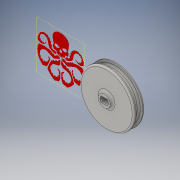
# Autodesk Inventor part: Wheel
Saved by Autodesk Inventor 2016 (Build 200138000, 138)
## iProperties
Created: 2017-09-08
Part Number: Wheel
Material: Generic
Document SubType Name: Modeling
Designer: student
Density: 1 g/cm^3
Appearance: Default
Author: student
Autodesk Inventor part; units mm, degrees
ref_plane "YZ Plane" through (0, 0, 0) normal (1, 0, 0) x (0, 1, 0)
ref_plane "XZ Plane" through (0, 0, 0) normal (0, 1, 0) x (-1, 0, 0)
ref_plane "XY Plane" through (0, 0, 0) normal (0, 0, 1) x (1, 0, 0)
sketch "Sketch8" plane through (0, 0, 0) normal (0, 0, 1) x (1, 0, 0)
  circle A0 centre (0, 0) radius 4.953
  dimension "d46" = 9.906
  constraints: 1 centre point, 1 coincident
  measures "d46" diameter of A0
extrude "Extrusion5" add sketch "Sketch8" along normal blind 2.032
sketch "Sketch9" plane through (0, 0, 0) normal (0, 0, -1) x (-1, 0, 0)
  circle A0 centre (0, 0) radius 22.479
  dimension "d49" = 44.958
  constraints: 1 centre point, 1 coincident
  measures "d49" diameter of A0
extrude "Extrusion6" add sketch "Sketch9" along normal blind 2.032
sketch "Sketch10" plane through (0, 0, -2.032) normal (0, 0, -1) x (-1, 0, 0)
  circle A0 centre (0, 0) radius 19.2405
  dimension "d52" = 38.481
  constraints: 1 centre point, 1 coincident
  measures "d52" diameter of A0
extrude "Extrusion7" add sketch "Sketch10" along normal blind 5.3086
sketch "Sketch11" plane through (0, 0, -7.3406) normal (0, 0, -1) x (-1, 0, 0)
  circle A0 centre (0, 0) radius 22.479
  dimension "d55" = 44.958
  constraints: 1 centre point, 1 coincident
  measures "d55" diameter of A0
extrude "Extrusion8" add sketch "Sketch11" along normal blind 2.032
fillet "Fillet1" radius 1.27 2 edges at (19.2405, 0, -2.032) (19.2405, 0, -7.3406)
sketch "Sketch12" plane through (0, 0, 2.032) normal (0, 0, 1) x (1, 0, 0)
  line L0 (2.5424, 2.413) -> (-2.5424, 2.413)
  line L1 (-2.5424, -2.413) -> (2.5424, -2.413)
  arc A0 (2.5424, -2.413) -> (2.5424, 2.413) centre (0, 0) ccw
  arc A1 (-2.5424, 2.413) -> (-2.5424, -2.413) centre (0, 0) ccw
  constraints: 4 end point, 4 point on circle, 2 centre point, 1 coincident, 1 horizontal, 1 parallel
fillet "Fillet2" radius 2.032 1 edges at (-4.953, 0, 0)
extrude "Extrusion9" cut sketch "Sketch12" against normal blind 5.4864
fillet "Fillet3" radius 1.27 2 edges at (22.479, 0, 0) (22.479, 0, -9.3726)
sketch "Sketch13" plane through (0, 0, -9.3726) normal (0, 0, -1) x (-1, 0, 0)
  line L0 (27.3817, 21.0767) -> (67.4327, 21.0767) construction
  line L1 (67.4327, 21.0767) -> (67.4327, -18.9549) construction
  line L2 (67.4327, -18.9549) -> (27.3817, -18.9549) construction
  line L3 (27.3817, -18.9549) -> (27.3817, 21.0767) construction
  point P0 (0, 0)
  constraints: 2 other
sketch "Sketch14" plane through (0, 0, -9.3726) normal (0, 0, -1) x (-1, 0, 0)
  arc A0 (-4.5923, 12.1139) -> (-4.8812, 11.9177) centre (-4.2357, 11.2781) ccw
  arc A1 (-4.5923, 12.1139) -> (-4.3633, 12.4084) centre (-4.944, 12.6237) ccw
  arc A2 (-4.3633, 12.4084) -> (-4.3916, 12.9039) centre (-4.944, 12.6237) ccw
  arc A3 (-4.8158, 14.8456) -> (-4.3916, 12.9039) centre (3.5016, 15.6455) ccw
  arc A4 (-4.8812, 17.2664) -> (-4.8158, 14.8456) centre (1.7367, 16.234) ccw
  arc A5 (-4.0539, 18.7211) -> (-4.8812, 17.2664) centre (-1.7423, 16.4438) ccw
  arc A6 (-1.5444, 20.1344) -> (-4.0539, 18.7211) centre (-0.3415, 15.0638) ccw
  arc A7 (1.4435, 20.0526) -> (-1.5444, 20.1344) centre (-0.2795, 11.7292) ccw
  arc A8 (3.8761, 18.5407) -> (1.4435, 20.0526) centre (0.0651, 15.1216) ccw
  arc A9 (4.5915, 16.9853) -> (3.8761, 18.5407) centre (1.7211, 16.6073) ccw
  arc A10 (4.4696, 14.7311) -> (4.5915, 16.9853) centre (-6.4235, 16.4508) ccw
  arc A11 (4.0007, 12.852) -> (4.4696, 14.7311) centre (-6.4235, 16.4508) ccw
  arc A12 (4.0007, 12.852) -> (4.3223, 12.0649) centre (4.673, 12.6674) ccw
  arc A13 (4.5575, 11.7797) -> (4.3223, 12.0649) centre (4.3186, 11.8222) ccw
  arc A14 (4.0277, 10.2165) -> (4.5575, 11.7797) centre (-0.8578, 12.7438) ccw
  arc A15 (3.6953, 10.042) -> (4.0277, 10.2165) centre (3.6694, 10.4951) ccw
  arc A16 (3.6953, 10.042) -> (2.643, 9.9968) centre (3.3355, 6.1474) ccw
  arc A17 (2.643, 9.9968) -> (2.1034, 9.7949) centre (2.7888, 8.7852) ccw
  arc A18 (2.1034, 9.7949) -> (2.0743, 9.6271) centre (2.1699, 9.6969) ccw
  arc A19 (2.3213, 9.5949) -> (2.0743, 9.6271) centre (2.1194, 9.0082) ccw
  arc A20 (2.4777, 9.5148) -> (2.3213, 9.5949) centre (2.1194, 9.0082) ccw
  arc A21 (2.2164, 8.7351) -> (2.4777, 9.5148) centre (-2.9872, 10.913) ccw
  arc A22 (1.5804, 8.3678) -> (2.2164, 8.7351) centre (-0.6752, 13.007) ccw
  line L0 (1.5804, 8.3678) -> (1.5804, 9.0749)
  line L1 (1.5804, 9.0749) -> (1.4748, 9.0749)
  line L2 (1.4748, 9.0749) -> (1.4748, 8.3179)
  line L3 (1.4748, 8.3179) -> (0.8106, 8.0671)
  line L4 (0.8106, 8.0671) -> (0.8106, 8.8752)
  line L5 (0.8106, 8.8752) -> (0.646, 8.8752)
  line L6 (0.646, 8.8752) -> (0.646, 7.9869)
  line L7 (0.646, 7.9869) -> (-0.0795, 7.7663)
  line L8 (-0.0795, 7.7663) -> (-0.0795, 8.7099)
  line L9 (-0.0795, 8.7099) -> (-0.2563, 8.7099)
  line L10 (-0.2563, 8.7099) -> (-0.2563, 7.7663)
  line L11 (-0.2563, 7.7663) -> (-0.9794, 7.9869)
  line L12 (-0.9794, 7.9869) -> (-0.9794, 8.8637)
  line L13 (-0.9794, 8.8637) -> (-1.1493, 8.8637)
  line L14 (-1.1493, 8.8637) -> (-1.1493, 8.0387)
  line L15 (-1.1493, 8.0387) -> (-1.7423, 8.2943)
  line L16 (-1.7423, 8.2943) -> (-1.8105, 9.0749)
  line L17 (-1.8105, 9.0749) -> (-1.9205, 9.0749)
  line L18 (-1.9205, 9.0749) -> (-1.8771, 8.3678)
  line L19 (-1.8771, 8.3678) -> (-1.9457, 8.3678)
  line L20 (-1.9457, 8.3678) -> (-2.5567, 8.7214)
  line L21 (-2.5567, 8.7214) -> (-2.8092, 9.5148)
  arc A23 (-2.6436, 9.6153) -> (-2.8092, 9.5148) centre (-2.615, 9.3813) ccw
  arc A24 (-2.6436, 9.6153) -> (-2.4007, 9.6567) centre (-2.6703, 10.5051) ccw
  arc A25 (-2.4007, 9.6567) -> (-2.4329, 9.7845) centre (-2.4862, 9.7031) ccw
  arc A26 (-2.4329, 9.7845) -> (-3.1333, 10.0284) centre (-3.3716, 8.2163) ccw
  arc A27 (-3.1333, 10.0284) -> (-3.3592, 10.044) centre (-3.3716, 8.2163) ccw
  line L22 (-3.3592, 10.044) -> (-4.0618, 10.044)
  arc A28 (-4.3765, 10.2165) -> (-4.0618, 10.044) centre (-4.0323, 10.4709) ccw
  arc A29 (-4.7223, 11.1859) -> (-4.3765, 10.2165) centre (-1.0099, 11.964) ccw
  arc A30 (-4.8812, 11.6735) -> (-4.7223, 11.1859) centre (3.9571, 14.2843) ccw
  line L23 (-4.8812, 11.6735) -> (-4.8812, 11.9177)
  line L24 (2.0532, 9.7172) -> (0.5491, 10.2165) construction
  arc A31 (0.5491, 10.2165) -> (0.6304, 10.4172) centre (0.1536, 10.4935) ccw
  arc A32 (0.6304, 10.4172) -> (-0.1679, 11.997) centre (-4.6953, 8.7178) ccw
  arc A33 (-0.1679, 11.997) -> (-0.9442, 10.5444) centre (5.3013, 8.14) ccw
  arc A34 (-0.9442, 10.5444) -> (-0.8343, 10.1434) centre (-0.5613, 10.4338) ccw
  arc A35 (-0.8343, 10.1434) -> (-0.5066, 10.055) centre (-0.5932, 10.3856) ccw
  arc A36 (-0.1679, 10.3284) -> (-0.5066, 10.055) centre (-0.0487, 9.8343) ccw
  arc A37 (0.1949, 10.0341) -> (-0.1679, 10.3284) centre (-0.22, 9.8934) ccw
  arc A38 (0.1949, 10.0341) -> (0.4536, 10.0933) centre (0.2807, 10.2541) ccw
  arc A39 (0.4536, 10.0933) -> (0.5491, 10.2165) centre (0.2539, 10.3467) ccw
  line L25 (-4.4858, 12.207) -> (-3.6366, 12.1139) construction
  line L26 (-3.6366, 12.1139) -> (-3.6366, 12.9376)
  arc A40 (-3.1333, 13.3967) -> (-3.6366, 12.9376) centre (-2.9549, 12.6957) ccw
  arc A41 (-2.4329, 13.3967) -> (-3.1333, 13.3967) centre (-2.7831, 12.3837) ccw
  arc A42 (-0.8681, 12.493) -> (-2.4329, 13.3967) centre (-4.3475, 8.2748) ccw
  arc A43 (-0.9794, 12.319) -> (-0.8681, 12.493) centre (-1.1724, 12.5651) ccw
  arc A44 (-2.3919, 11.5856) -> (-0.9794, 12.319) centre (-4.1175, 16.6352) ccw
  arc A45 (-2.7121, 11.6161) -> (-2.3919, 11.5856) centre (-2.4563, 12.6034) ccw
  arc A46 (-3.6366, 12.1139) -> (-2.7121, 11.6161) centre (-2.1218, 13.8197) ccw
  arc A47 (0.5687, 12.4767) -> (-0.8681, 12.493) centre (-0.4902, -17.6157) ccw construction
  arc A48 (2.4024, 13.4555) -> (0.5687, 12.4767) centre (3.4409, 9.303) ccw
  arc A49 (3.3201, 12.9782) -> (2.4024, 13.4555) centre (2.558, 12.6338) ccw
  arc A50 (3.3201, 12.1139) -> (3.3201, 12.9782) centre (-1.9015, 12.5461) ccw
  arc A51 (2.4024, 11.6018) -> (3.3201, 12.1139) centre (1.2914, 14.6713) ccw
  arc A52 (1.9298, 11.6547) -> (2.4024, 11.6018) centre (2.2524, 12.4001) ccw
  arc A53 (0.9974, 12.0851) -> (1.9298, 11.6547) centre (3.0242, 15.2512) ccw
  arc A54 (0.5687, 12.4767) -> (0.9974, 12.0851) centre (1.3606, 12.913) ccw
  circle A55 centre (0, 0) radius 6.985 projected
  constraints: 116 point on circle, 55 centre point, 54 end point, 8 perpendicular, 4 concentric, 4 tangent, 3 parallel, 3 vertical, 2 horizontal, 2 point on line
sketch "Sketch15" plane through (0, 0, -9.3726) normal (0, 0, -1) x (-1, 0, 0)
  arc A0 (3.2835, -4.4275) -> (5.1961, -4.1737) centre (3.5629, 0.8007) ccw
  arc A1 (0.4839, -2.9385) -> (3.2835, -4.4275) centre (8.7601, 9.2457) ccw
  arc A2 (-0.1806, -1.9597) -> (0.4839, -2.9385) centre (2.084, -1.1373) ccw
  arc A3 (-0.5458, -0.6157) -> (-0.1806, -1.9597) centre (4.987, 0.1664) ccw
  arc A4 (-0.5458, -0.6157) -> (-0.8315, 0.7143) centre (-15.1738, -3.0619) ccw
  arc A5 (-0.8315, 0.7143) -> (-1.4332, 2.0501) centre (-8.2084, -1.805) ccw
  arc A6 (-1.4332, 2.0501) -> (-2.2365, 2.8199) centre (-4.9322, -0.797) ccw
  arc A7 (-2.2365, 2.8199) -> (-3.2699, 3.2592) centre (-4.155, -0.2579) ccw
  arc A8 (-3.2699, 3.2592) -> (-4.155, 3.322) centre (-3.9447, 0.015) ccw
  arc A9 (-4.155, 3.322) -> (-4.5262, 3.2773) centre (-4.2753, 2.7578) ccw
  line L0 (-4.5262, 3.2773) -> (-4.5262, 3.0954)
  line L1 (-4.5262, 3.0954) -> (-5.1612, 2.7808)
  line L2 (-5.1612, 2.7808) -> (-5.3504, 2.9381)
  line L3 (-5.3504, 2.9381) -> (-5.8649, 2.5462)
  line L4 (-5.8649, 2.5462) -> (-5.7115, 2.3447)
  line L5 (-5.7115, 2.3447) -> (-6.0462, 1.7651)
  line L6 (-6.0462, 1.7651) -> (-6.3981, 1.8504)
  line L7 (-6.3981, 1.8504) -> (-6.6074, 1.233)
  line L8 (-6.6074, 1.233) -> (-6.3099, 1.1609)
  line L9 (-6.3099, 1.1609) -> (-6.3099, 0.5174)
  line L10 (-6.3099, 0.5174) -> (-6.6247, 0.3442)
  line L11 (-6.6247, 0.3442) -> (-6.5027, -0.205)
  line L12 (-6.5027, -0.205) -> (-6.1475, -0.1502)
  line L13 (-6.1475, -0.1502) -> (-5.815, -0.5868)
  line L14 (-5.815, -0.5868) -> (-6.0243, -0.9491)
  line L15 (-6.0243, -0.9491) -> (-5.5877, -1.3807)
  line L16 (-5.5877, -1.3807) -> (-5.3371, -1.1043)
  line L17 (-5.3371, -1.1043) -> (-4.8104, -1.3272)
  line L18 (-4.8104, -1.3272) -> (-4.8104, -1.7164)
  line L19 (-4.8104, -1.7164) -> (-4.243, -1.7164)
  line L20 (-4.243, -1.7164) -> (-4.243, -1.6019)
  line L21 (-4.243, -1.6019) -> (-3.6128, -1.4337)
  line L22 (-3.6128, -1.4337) -> (-3.4189, -1.6883)
  line L23 (-3.4189, -1.6883) -> (-2.9185, -1.4128)
  line L24 (-2.9185, -1.4128) -> (-2.9299, -1.1484)
  line L25 (-2.9299, -1.1484) -> (-2.4798, -0.8613)
  line L26 (-2.4798, -0.8613) -> (-2.3555, -0.9139)
  line L27 (-2.3555, -0.9139) -> (-2.0395, -0.5654)
  line L28 (-2.0395, -0.5654) -> (-2.0395, -1.1373)
  arc A10 (-3.9447, -2.5482) -> (-2.0395, -1.1373) centre (-11.1321, 9.1493) ccw
  arc A11 (-5.6195, -2.8996) -> (-3.9447, -2.5482) centre (-5.892, 2.5664) ccw
  line L29 (-5.6195, -2.8996) -> (-6.0462, -2.8996)
  arc A12 (-6.0462, -2.8996) -> (-7.6246, -2.104) centre (-9.4191, -7.6278) ccw
  arc A13 (-7.9176, -1.805) -> (-7.6246, -2.104) centre (-7.5271, -1.7154) ccw
  line L30 (-7.9176, -1.805) -> (-7.9176, 0.015)
  arc A14 (-6.1475, 3.7162) -> (-7.9176, 0.015) centre (7.5851, -5.1251) ccw
  line L31 (-6.1475, 3.7162) -> (-3.8586, 4.7333)
  line L32 (-3.8586, 4.7333) -> (-2.4177, 4.7333)
  line L33 (-2.4177, 4.7333) -> (-2.4177, 4.5428)
  arc A15 (-1.7039, 4.3356) -> (-2.4177, 4.5428) centre (-2.3399, 3.4779) ccw
  line L34 (-1.7039, 4.3356) -> (-1.4454, 4.5033)
  line L35 (-1.4454, 4.5033) -> (-0.7022, 4.1202)
  line L36 (-0.7022, 4.1202) -> (-0.7088, 3.9183)
  line L37 (-0.7088, 3.9183) -> (-0.7372, 3.9192)
  line L38 (-0.7372, 3.9192) -> (-0.7372, 3.7637)
  arc A16 (-0.1806, 3.2313) -> (-0.7372, 3.7637) centre (-1.0541, 2.8751) ccw
  line L39 (-0.1806, 3.2313) -> (0.1939, 3.3306)
  line L40 (0.1939, 3.3306) -> (0.6393, 2.6323)
  line L41 (0.6393, 2.6323) -> (0.5063, 2.4021)
  arc A17 (0.7504, 1.7651) -> (0.5063, 2.4021) centre (-0.8029, 1.5351) ccw
  line L42 (0.7504, 1.7651) -> (1.2473, 1.7866)
  line L43 (1.2473, 1.7866) -> (1.4586, 0.9351)
  line L44 (1.4586, 0.9351) -> (1.1292, 0.655)
  arc A18 (1.3529, -0.1502) -> (1.1292, 0.655) centre (-1.2589, -0.4423) ccw
  line L45 (1.3529, -0.1502) -> (1.8859, -0.1776)
  line L46 (1.8859, -0.1776) -> (2.1272, -1.0048)
  line L47 (2.1272, -1.0048) -> (1.7779, -1.3807)
  arc A19 (1.7779, -1.3807) -> (2.2899, -2.4143) centre (4.5818, -0.6354) ccw
  arc A20 (2.2899, -2.4143) -> (2.6824, -2.5729) centre (2.7029, -1.9572) ccw
  line L48 (2.6824, -2.5729) -> (4.4075, -2.6475)
  line L49 (4.4075, -2.6475) -> (5.1961, -4.1737)
  line L50 (7.5643, -5.1725) -> (7.5643, -5.932)
  line L51 (7.5643, -5.932) -> (4.3041, -7.4715)
  arc A21 (3.7086, -7.7018) -> (4.3041, -7.4715) centre (2.414, -3.4692) ccw
  line L52 (3.7086, -7.7018) -> (3.5844, -7.7018)
  line L53 (3.5844, -7.7018) -> (3.1371, -7.7018)
  line L54 (3.1371, -7.7018) -> (2.6252, -7.5333)
  line L55 (2.6252, -7.5333) -> (1.3343, -6.9528)
  line L56 (1.3343, -6.9528) -> (0.2407, -6.493)
  line L57 (0.2407, -6.493) -> (-0.8589, -6.0549)
  line L58 (-0.8589, -6.0549) -> (-1.92, -5.6657)
  arc A22 (-1.92, -5.6657) -> (-2.4864, -5.4761) centre (-5.5219, -15.4849) ccw
  arc A23 (-2.4864, -5.4761) -> (-2.9185, -5.4906) centre (-2.6811, -6.1183) ccw
  line L59 (-2.9185, -5.4906) -> (-3.5158, -5.6488)
  arc A24 (-3.5158, -5.6488) -> (-4.4656, -6.0026) centre (-2.1845, -10.6746) ccw
  arc A25 (-4.4656, -6.0026) -> (-5.4624, -6.7447) centre (-2.9896, -9.0256) ccw
  arc A26 (-5.4624, -6.7447) -> (-6.1419, -7.6176) centre (-0.5922, -11.237) ccw
  arc A27 (-6.1419, -7.6176) -> (-6.5244, -8.4628) centre (-3.5921, -9.2805) ccw
  line L60 (-6.5244, -8.4628) -> (-6.3981, -8.5607)
  line L61 (-6.3981, -8.5607) -> (-6.3867, -8.5758)
  line L62 (-6.3867, -8.5758) -> (-6.3867, -9.472)
  line L63 (-6.3867, -9.472) -> (-6.6889, -9.6063)
  line L64 (-6.6889, -9.6063) -> (-6.5428, -10.4465)
  line L65 (-6.5428, -10.4465) -> (-6.1636, -10.426)
  line L66 (-6.1636, -10.426) -> (-5.7472, -11.1091)
  line L67 (-5.7472, -11.1091) -> (-6.0462, -11.4732)
  line L68 (-6.0462, -11.4732) -> (-6.0422, -11.5485)
  line L69 (-6.0422, -11.5485) -> (-5.8204, -11.8397)
  line L70 (-5.8204, -11.8397) -> (-5.4624, -12.164)
  line L71 (-5.4624, -12.164) -> (-5.1506, -11.8813)
  line L72 (-5.1506, -11.8813) -> (-4.4468, -12.1772)
  line L73 (-4.4468, -12.1772) -> (-4.4286, -12.1877)
  line L74 (-4.4286, -12.1877) -> (-4.4286, -12.7163)
  line L75 (-4.4286, -12.7163) -> (-4.0845, -12.861)
  line L76 (-4.0845, -12.861) -> (-3.6564, -12.8749)
  line L77 (-3.6564, -12.8749) -> (-3.5921, -12.452)
  line L78 (-3.5921, -12.452) -> (-2.8009, -12.3239)
  line L79 (-2.8009, -12.3239) -> (-2.5348, -12.8074)
  arc A28 (-1.811, -12.5219) -> (-2.5348, -12.8074) centre (-1.06, -15.4866) ccw
  line L80 (-1.811, -12.5219) -> (-1.92, -12.1104)
  line L81 (-1.92, -12.1104) -> (-1.3341, -11.5793)
  line L82 (-1.3341, -11.5793) -> (-0.9338, -11.8105)
  line L83 (-0.9338, -11.8105) -> (-0.5458, -11.1763)
  line L84 (-0.5458, -11.1763) -> (-0.6954, -11.0004)
  line L85 (-0.6954, -11.0004) -> (-0.5033, -10.2652)
  line L86 (-0.5033, -10.2652) -> (-0.4907, -10.2446)
  line L87 (-0.4907, -10.2446) -> (-0.1038, -10.2446)
  line L88 (-0.1038, -10.2446) -> (-0.1038, -9.6527)
  line L89 (-0.1038, -9.6527) -> (-0.08, -9.6421)
  line L90 (-0.08, -9.6421) -> (-0.08, -9.4656)
  line L91 (-0.08, -9.4656) -> (-0.4176, -9.4345)
  line L92 (-0.4176, -9.4345) -> (-0.4315, -9.1783)
  line L93 (-0.4315, -9.1783) -> (-0.4509, -8.5724)
  line L94 (-0.4509, -8.5724) -> (-0.4114, -8.5366)
  arc A29 (-0.4114, -8.5366) -> (-0.313, -8.2973) centre (-0.6137, -8.3135) ccw
  line L95 (-0.313, -8.2973) -> (-0.3818, -8.0376)
  arc A30 (-0.3818, -8.0376) -> (-0.3535, -8.0006) centre (-0.3915, -8.0009) ccw
  line L96 (-0.3535, -8.0006) -> (-0.3091, -7.9992)
  line L97 (-0.3091, -7.9992) -> (-0.2464, -8.0376)
  line L98 (-0.2464, -8.0376) -> (0.0779, -8.4939)
  line L99 (0.0779, -8.4939) -> (0.2584, -8.8218)
  line L100 (0.2584, -8.8218) -> (0.4805, -9.3217)
  line L101 (0.4805, -9.3217) -> (0.555, -9.5125)
  arc A31 (0.5651, -10.0803) -> (0.555, -9.5125) centre (-0.2079, -9.8101) ccw
  line L102 (0.5651, -10.0803) -> (0.3403, -10.7634)
  arc A32 (-0.6137, -13.0465) -> (0.3403, -10.7634) centre (-14.7776, -5.7874) ccw
  line L103 (-0.6137, -13.0465) -> (-1.5565, -15.0218)
  line L104 (-1.5565, -15.0218) -> (-4.3183, -15.5766)
  arc A33 (-4.6984, -15.5492) -> (-4.3183, -15.5766) centre (-4.4588, -14.8773) ccw
  line L105 (-4.6984, -15.5492) -> (-5.0363, -15.2042)
  line L106 (-5.0363, -15.2042) -> (-5.6414, -14.4924)
  line L107 (-5.6414, -14.4924) -> (-6.443, -13.5208)
  line L108 (-6.443, -13.5208) -> (-6.9167, -12.8281)
  arc A34 (-7.5918, -11.3442) -> (-6.9167, -12.8281) centre (-3.0056, -10.1532) ccw
  line L109 (-7.5918, -11.3442) -> (-7.875, -10.2829)
  line L110 (-7.875, -10.2829) -> (-8.0596, -9.2617)
  arc A35 (-8.1089, -6.5488) -> (-8.0596, -9.2617) centre (0.2886, -7.7531) ccw
  line L111 (-8.1089, -6.5488) -> (-7.9387, -5.4296)
  arc A36 (-7.8338, -5.1251) -> (-7.9387, -5.4296) centre (-7.0543, -5.564) ccw
  line L112 (-7.8338, -5.1251) -> (-7.6559, -4.6046)
  arc A37 (-7.5758, -4.4522) -> (-7.6559, -4.6046) centre (-7.1279, -4.785) ccw
  arc A38 (-7.0991, -3.9741) -> (-7.5758, -4.4522) centre (-5.6999, -5.846) ccw
  arc A39 (-6.4305, -3.6885) -> (-7.0991, -3.9741) centre (-6.1764, -5.2085) ccw
  line L113 (-6.4305, -3.6885) -> (-5.3201, -3.5575)
  line L114 (-5.3201, -3.5575) -> (-4.5402, -3.4833)
  line L115 (-4.5402, -3.4833) -> (-3.7103, -3.4593)
  line L116 (-3.7103, -3.4593) -> (-2.6811, -3.4927)
  arc A40 (-0.7615, -3.923) -> (-2.6811, -3.4927) centre (-2.8513, -8.7481) ccw
  line L117 (-0.7615, -3.923) -> (-0.5362, -3.6173)
  line L118 (-0.5362, -3.6173) -> (0.2886, -3.7702)
  line L119 (0.2886, -3.7702) -> (0.2962, -4.0313)
  line L120 (0.2962, -4.0313) -> (0.8472, -4.2846)
  line L121 (0.8472, -4.2846) -> (1.1855, -4.0543)
  line L122 (1.1855, -4.0543) -> (1.8867, -4.4104)
  line L123 (1.8867, -4.4104) -> (1.9257, -4.8204)
  line L124 (1.9257, -4.8204) -> (2.4828, -5.1795)
  line L125 (2.4828, -5.1795) -> (2.9173, -4.8648)
  line L126 (2.9173, -4.8648) -> (3.5786, -5.2695)
  line L127 (3.5786, -5.2695) -> (3.5786, -5.6113)
  line L128 (-2.5424, -2.413) -> (2.5424, -2.413) projected
  arc A41 (3.5786, -5.6113) -> (3.9297, -5.7574) centre (3.7846, -5.6113) ccw
  line L129 (3.9297, -5.7574) -> (4.7177, -5.2829)
  line L130 (4.7177, -5.2829) -> (6.0013, -4.4538)
  line L131 (6.0013, -4.4538) -> (7.5643, -5.1725)
  line L132 (7.9421, -6.4366) -> (7.9421, -9.0223)
  line L133 (7.9421, -9.0223) -> (6.696, -10.4756)
  line L134 (6.696, -10.4756) -> (4.33, -10.9452)
  arc A42 (4.33, -10.9452) -> (3.3565, -11.1775) centre (6.8671, -23.7299) ccw
  arc A43 (3.3565, -11.1775) -> (2.4487, -11.756) centre (3.8557, -12.9623) ccw
  line L135 (2.4487, -11.756) -> (1.9257, -12.366)
  line L136 (1.9257, -12.366) -> (1.5707, -12.8281)
  line L137 (1.5707, -12.8281) -> (1.3415, -13.2026)
  arc A44 (1.3415, -13.2026) -> (0.9988, -13.9423) centre (4.362, -15.051) ccw
  arc A45 (0.9988, -13.9423) -> (0.8819, -14.509) centre (3.3954, -14.7324) ccw
  line L138 (0.8819, -14.509) -> (0.8819, -15.111)
  line L139 (0.8819, -15.111) -> (0.9417, -15.6179)
  line L140 (0.9417, -15.6179) -> (1.0973, -15.6569)
  line L141 (1.0973, -15.6569) -> (1.5455, -16.4346)
  line L142 (1.5455, -16.4346) -> (1.386, -16.6692)
  line L143 (1.386, -16.6692) -> (1.8215, -17.2564)
  line L144 (1.8215, -17.2564) -> (2.1056, -17.0926)
  line L145 (2.1056, -17.0926) -> (2.7852, -17.5546)
  line L146 (2.7852, -17.5546) -> (2.6938, -17.9199)
  line L147 (2.6938, -17.9199) -> (3.411, -18.2057)
  line L148 (3.411, -18.2057) -> (3.6008, -17.8319)
  line L149 (3.6008, -17.8319) -> (4.3791, -17.8319)
  line L150 (4.3791, -17.8319) -> (4.6085, -18.2485)
  line L151 (4.6085, -18.2485) -> (5.2754, -18.0705)
  line L152 (5.2754, -18.0705) -> (5.2258, -17.6504)
  line L153 (5.2258, -17.6504) -> (5.8027, -17.2226)
  line L154 (5.8027, -17.2226) -> (6.1912, -17.4867)
  line L155 (6.1912, -17.4867) -> (6.6837, -16.9037)
  line L156 (6.6837, -16.9037) -> (6.3995, -16.6049)
  line L157 (6.3995, -16.6049) -> (6.3968, -16.5111)
  line L158 (6.3968, -16.5111) -> (6.6338, -15.984)
  line L159 (6.6338, -15.984) -> (6.6502, -15.9185)
  line L160 (6.6502, -15.9185) -> (7.1269, -15.8931)
  line L161 (7.1269, -15.8931) -> (7.1406, -15.2248)
  line L162 (7.1406, -15.2248) -> (6.9627, -15.2191)
  line L163 (6.9627, -15.2191) -> (6.7283, -14.4755)
  line L164 (6.7283, -14.4755) -> (7.0355, -14.1833)
  line L165 (7.0355, -14.1833) -> (6.7436, -13.653)
  line L166 (6.7436, -13.653) -> (6.4838, -13.6999)
  line L167 (6.4838, -13.6999) -> (6.023, -13.1231)
  line L168 (6.023, -13.1231) -> (6.056, -12.8281)
  line L169 (6.056, -12.8281) -> (5.8027, -12.5111)
  line L170 (5.8027, -12.5111) -> (5.8027, -12.4849)
  arc A46 (6.5416, -12.6272) -> (5.8027, -12.4849) centre (5.8027, -14.4742) ccw
  arc A47 (7.2608, -13.1405) -> (6.5416, -12.6272) centre (5.8494, -14.3575) ccw
  line L171 (7.2608, -13.1405) -> (7.8493, -13.823)
  line L172 (7.8493, -13.823) -> (7.8493, -17.5782)
  line L173 (7.8493, -17.5782) -> (7.7821, -17.775)
  line L174 (7.7821, -17.775) -> (7.7903, -17.8442)
  line L175 (7.7903, -17.8442) -> (7.6135, -18.3614)
  line L176 (7.6135, -18.3614) -> (7.4435, -18.7881)
  line L177 (7.4435, -18.7881) -> (7.2989, -19.1098)
  line L178 (7.2989, -19.1098) -> (7.0975, -19.5575)
  line L179 (7.0975, -19.5575) -> (6.9116, -19.9237)
  line L180 (6.9116, -19.9237) -> (3.9329, -20.8084)
  arc A48 (3.7623, -20.7871) -> (3.9329, -20.8084) centre (3.8719, -20.6031) ccw
  line L181 (3.7623, -20.7871) -> (2.7395, -20.2369)
  line L182 (2.7395, -20.2369) -> (1.9635, -19.6652)
  line L183 (1.9635, -19.6652) -> (1.3343, -19.1098)
  line L184 (1.3343, -19.1098) -> (0.8819, -18.6587)
  line L185 (0.8819, -18.6587) -> (0.4761, -18.2541)
  line L186 (0.4761, -18.2541) -> (0.0411, -17.7846)
  line L187 (0.0411, -17.7846) -> (-0.2464, -17.4867)
  line L188 (-0.2464, -17.4867) -> (-0.4931, -17.1964)
  line L189 (-0.4931, -17.1964) -> (-0.6014, -17.0609)
  line L190 (-0.6014, -17.0609) -> (-0.7084, -16.9037)
  line L191 (-0.7084, -16.9037) -> (-0.8678, -16.6888)
  arc A49 (-1.0002, -16.4421) -> (-0.8678, -16.6888) centre (-0.0917, -16.1133) ccw
  arc A50 (-1.0851, -16.1746) -> (-1.0002, -16.4421) centre (2.3004, -15.2478) ccw
  line L192 (-1.0851, -16.1746) -> (-1.0944, -16.0009)
  arc A51 (-1.0002, -15.676) -> (-1.0944, -16.0009) centre (-0.5812, -15.9735) ccw
  line L193 (-1.0002, -15.676) -> (-0.9119, -15.4177)
  line L194 (-0.9119, -15.4177) -> (-0.7615, -14.905)
  line L195 (-0.7615, -14.905) -> (-0.5744, -14.3575)
  line L196 (-0.5744, -14.3575) -> (-0.3563, -13.7629)
  line L197 (-0.3563, -13.7629) -> (-0.1997, -13.363)
  line L198 (-0.1997, -13.363) -> (-0.0401, -12.9622)
  line L199 (-0.0401, -12.9622) -> (0.144, -12.5219)
  line L200 (0.144, -12.5219) -> (0.5096, -11.7881)
  line L201 (0.5096, -11.7881) -> (0.8303, -11.1729)
  line L202 (0.8303, -11.1729) -> (0.9766, -10.9339)
  line L203 (0.9766, -10.9339) -> (1.2443, -10.4916)
  arc A52 (1.2443, -10.4916) -> (1.3468, -10.0338) centre (0.6142, -10.1102) ccw
  line L204 (1.3468, -10.0338) -> (1.6951, -9.7469)
  line L205 (1.6951, -9.7469) -> (1.8633, -9.8761)
  line L206 (1.8633, -9.8761) -> (2.4876, -9.5538)
  line L207 (2.4876, -9.5538) -> (2.4828, -9.0981)
  line L208 (2.4828, -9.0981) -> (3.329, -8.8187)
  line L209 (3.329, -8.8187) -> (3.6719, -9.0822)
  line L210 (3.6719, -9.0822) -> (4.3682, -8.8035)
  line L211 (4.3682, -8.8035) -> (4.3682, -8.3172)
  line L212 (4.3682, -8.3172) -> (5.179, -7.9569)
  line L213 (5.179, -7.9569) -> (5.5306, -8.2751)
  line L214 (5.5306, -8.2751) -> (5.7467, -8.1791)
  arc A53 (5.7467, -8.1791) -> (6.442, -7.5512) centre (5.1352, -6.8031) ccw
  line L215 (6.442, -7.5512) -> (6.9886, -6.7825)
  line L216 (6.9886, -6.7825) -> (7.9421, -6.4366)
  point P0 (0, 0)
  constraints: 432 end point, 109 point on circle, 54 centre point, 49 parallel, 34 perpendicular, 32 tangent, 16 point on line, 6 vertical, 2 horizontal
body "Solid2"
